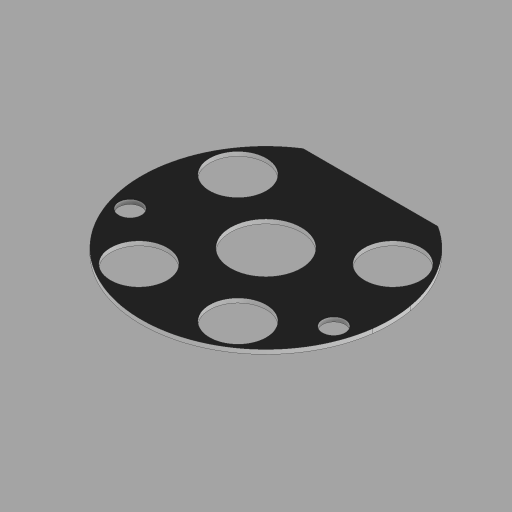
# Autodesk Inventor part: vverh
Saved by Autodesk Inventor 2024.2 (Build 282272000, 272)
## iProperties
Created: 2024-03-11
Part Number: vverh
Material: Типовые
Document SubType Name: Modeling
Designer: Fedor Orlov
Density: 1 g/cm^3
Appearance: По умолчанию
Author: Fedor Orlov
Autodesk Inventor part; units mm, degrees
ref_plane "YZ Plane" through (0, 0, 0) normal (1, 0, 0) x (0, 1, 0)
ref_plane "XZ Plane" through (0, 0, 0) normal (0, 1, 0) x (-1, 0, 0)
ref_plane "XY Plane" through (0, 0, 0) normal (0, 0, 1) x (1, 0, 0)
sketch "Эскиз1" plane through (0, 0, 0) normal (0, 1, 0) x (-1, 0, 0)
  arc A0 (46.7842, -80.4226) -> (85.3343, -22.1214) centre (-1.3087, -6.7268) ccw
  spline S0 degree 3 poles (85.3343, -22.1214) (85.7228, -19.9347) (86.0863, -17.3865) (86.5105, -12.698) (86.6278, -10.6493) (86.6714, -8.5984) (86.715, -6.5474) (86.685, -4.4956) (86.4606, 0.2067) (86.2058, 2.768) (85.9106, 4.9693) knots -3.249933 -3.249933 -3.249933 -3.249933 -2.410881 -2.410881 -1.809443 -1.809443 -1.809443 -1.208005 -1.208005 -0.368953 -0.368953 -0.368953 -0.368953
  arc A1 (85.9106, 4.9693) -> (-88.528, 4.9693) centre (-1.3087, -6.7268) ccw
  spline S1 degree 3 poles (-88.528, 4.9693) (-88.8231, 2.768) (-89.078, 0.2067) (-89.3023, -4.4956) (-89.3324, -6.5474) (-89.2888, -8.5984) (-89.2451, -10.6493) (-89.1279, -12.698) (-88.7037, -17.3865) (-88.3402, -19.9347) (-87.9517, -22.1214) knots -3.249933 -3.249933 -3.249933 -3.249933 -2.410881 -2.410881 -1.809443 -1.809443 -1.809443 -1.208005 -1.208005 -0.368953 -0.368953 -0.368953 -0.368953
  arc A2 (-87.9517, -22.1214) -> (-49.4016, -80.4226) centre (-1.3087, -6.7268) ccw
  line L0 (-48.3085, -80.7477) -> (45.6912, -80.7477)
  arc A3 (-49.4016, -80.4226) -> (-48.3085, -80.7477) centre (-48.3085, -78.7477) ccw
  arc A4 (45.6912, -80.7477) -> (46.7842, -80.4226) centre (45.6912, -78.7477) ccw
  circle A5 centre (53.4633, -41.7268) radius 20
  circle A6 centre (-56.0807, -41.7268) radius 20
  circle A7 centre (-36.3087, 48.0452) radius 20
  circle A8 centre (33.6913, 48.0452) radius 20
  circle A9 centre (-1.3087, -6.7268) radius 25
  circle A10 centre (70.6913, 17.2732) radius 3.25 construction
  circle A11 centre (-73.3087, 17.2732) radius 3.25 construction
  circle A12 centre (70.6913, 17.2732) radius 8
  circle A13 centre (-73.3087, 17.2732) radius 8
  point P0 (0, 0)
  dimension "d0" = 16
  dimension "d1" = 16
  constraints: 14 centre point, 10 point on circle, 2 coincident, 2 end point, 4 other
  measures "d0" diameter of A12
  measures "d1" diameter of A13
extrude "Выдавливание1" add sketch "Эскиз1" along normal blind 3
